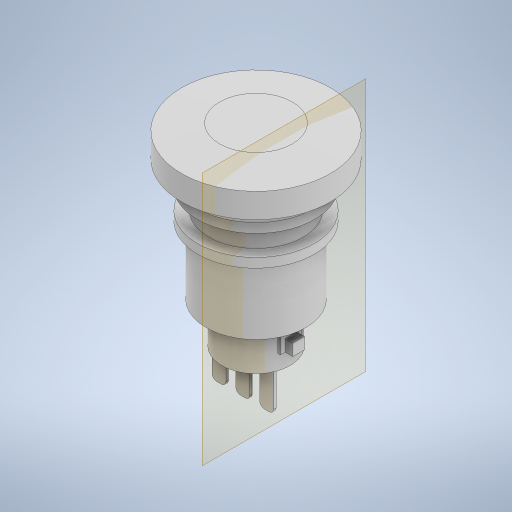
# Autodesk Inventor part: Co-1-01-eStopButton
Saved by Autodesk Inventor 2024 (Build 280153000, 153)
## iProperties
Created: 2023-02-23
Part Number: Co-1-01-eStopButton
Material: Generic
Document SubType Name: Modeling
Designer: t205b
Density: 1 g/cm^3
Appearance: Default
Author: t205b
Autodesk Inventor part; units mm, degrees
ref_plane "XZ Plane" through (0, 0, 0) normal (0, 1, 0) x (-1, 0, 0)
ref_plane "XY Plane" through (0, 0, 0) normal (0, 0, 1) x (1, 0, 0)
sketch "Sketch1" plane through (0, 0, 0) normal (0, 0, 1) x (1, 0, 0)
  line L0 (0, 20.0573) -> (0, -21.2213)
  line L1 (0, -21.2213) -> (-7.3, -21.2213)
  line L2 (-7.3, -21.2213) -> (-7.3, -12.5213)
  line L3 (-7.3, -12.5213) -> (-10.65, -12.5213)
  line L4 (-10.65, 1.9287) -> (-12.425, 1.9287)
  line L5 (-12.425, 1.9287) -> (-12.425, 3.9287)
  line L6 (-12.425, 3.9287) -> (-10.1, 3.9287)
  line L7 (-10.1, 3.9287) -> (-10.1, 8.4287)
  line L8 (-10.1, 8.4287) -> (-12.5, 8.4287)
  line L9 (-12.5, 8.4287) -> (-12.5, 10.4287)
  line L10 (-12.5, 10.4287) -> (-15.9, 13.3766)
  line L11 (-15.9, 13.3766) -> (-15.9, 18.6266)
  line L12 (0, 23.9493) -> (0, -31.6262)
  line L13 (-10.65, -12.5213) -> (-10.65, 1.9287)
  line L14 (-15.9, 18.6266) -> (-7.775, 20.0573)
  line L15 (-7.775, 20.0573) -> (0, 20.0573)
  point P0 (0, 0)
  point P1 (-10.1, 6.1787)
  point P2 (-10.65, -5.2963)
  dimension "d2" = 31.8
  dimension "d3" = 25
  dimension "d5" = 20.2
  dimension "d6" = 24.85
  dimension "d9" = 14.6
  dimension "d10" = 8.7
  dimension "d13" = 2
  dimension "d14" = 4.5
  dimension "d15" = 4.5
  dimension "d16" = 2
  dimension "d17" = 5.25
  dimension "d19" = 21.3
  dimension "d20" = 14.45
  dimension "d21" = 15.55
  dimension "d22" = 8.25
  constraints: 32 end point, 9 perpendicular, 3 point on line, 2 midpoint, 2 vertical, 1 parallel, 1 other
  measures "d2" diameter of L11 L12
  measures "d3" diameter of L9 L12
  measures "d5" diameter of L7 L12
  measures "d6" diameter of L5 L12
  measures "d9" diameter of L2 L12
  measures "d10" distance of L1.end L2.end
  measures "d13" distance of L4.end L5.end
  measures "d14" distance of L6.end L7.end
  measures "d15" distance of L9.end L10.end
  measures "d16" distance of L8.end L9.end
  measures "d17" distance of L10.end L11.end
  measures "d19" diameter of point (-10.65, -5.296) L12
  measures "d20" distance of L3.end L4.start
  measures "d21" diameter of L14.end L12
  measures "d22" distance of L11.end L14.end
revolve "Revolution1" add sketch "Sketch1" angle 360 about axis through (0, 23.9493, 0) along (0, -1, 0)
sketch "Sketch2" plane through (0, -21.2213, 0) normal (0, -1, 0) x (1, 0, 0)
  line L0 (6.6, 2.8) -> (3.6, 2.8)
  line L1 (3.6, 2.8) -> (3.6, 2.3)
  line L2 (3.6, 2.3) -> (6.6, 2.3)
  line L3 (6.6, 2.3) -> (6.6, 2.8)
  line L4 (1.5, 2.8) -> (-1.5, 2.8)
  line L5 (-1.5, 2.8) -> (-1.5, 2.3)
  line L6 (-1.5, 2.3) -> (1.5, 2.3)
  line L7 (1.5, 2.3) -> (1.5, 2.8)
  line L8 (-3.6, 2.8) -> (-6.6, 2.8)
  line L9 (-6.6, 2.8) -> (-6.6, 2.3)
  line L10 (-6.6, 2.3) -> (-3.6, 2.3)
  line L11 (-3.6, 2.3) -> (-3.6, 2.8)
  circle A0 centre (0, 0) radius 7.3 projected
  point P0 (0, 0)
  dimension "d23" = 0.5
  dimension "d24" = 3
  dimension "d25" = 2.1
  dimension "d26" = 2.1
  dimension "d29" = 14.6
  dimension "d31" = 2.8
  dimension "d32" = 1.5
  constraints: 24 end point, 6 parallel, 4 point on line, 3 horizontal, 3 perpendicular, 2 collinear
  measures "d23" distance of L0.end L1.end
  measures "d24" distance of L1.end L2.end
  measures "d25" distance between parallel lines of L1 L7
  measures "d26" distance between parallel lines of L5 L11
  measures "d29" diameter of A0
  measures "d31" distance from line of L4 A0.centre
  measures "d32" distance from line of point (0, 0) L7
extrude "Extrusion1" add sketch "Sketch2" along normal blind 8 contours L3 L2 L1 L0 | L7 L6 L5 L4 | L11 L10 L9 L8
fillet "Fillet1" radius 1 6 edges at (6.6, -29.2213, 2.55) (3.6, -29.2213, 2.55) (-6.6, -29.2213, 2.55) (-3.6, -29.2213, 2.55) (-1.5, -29.2213, 2.55) (1.5, -29.2213, 2.55)
ref_plane "Work Plane1" through (6, 0, 0) normal (1, 0, 0) x (0, 1, 0)
sketch "Sketch3" plane through (6, 0, 0) normal (1, 0, 0) x (0, 1, 0)
  line L0 (-12.5213, 7.3) -> (-12.5213, -7.3) projected
  line L1 (-12.5213, 2.25) -> (-18.0213, 2.25)
  line L2 (-18.0213, 2.25) -> (-18.0213, -2.25)
  line L3 (-18.0213, -2.25) -> (-12.5213, -2.25)
  line L4 (-12.5213, -2.25) -> (-12.5213, 2.25)
  line L5 (-39.077, 0) -> (29.913, 0) projected
  point P0 (0, 0)
  dimension "d37" = 4.5
  dimension "d38" = 5.5
  dimension "d39" = 2.25
  constraints: 8 end point, 2 parallel, 1 horizontal, 1 perpendicular, 1 point on line
  measures "d37" distance of L1.end L2.end
  measures "d38" distance of L2.end L3.end
  measures "d39" distance between parallel lines of L5 L3
extrude "Extrusion2" add sketch "Sketch3" along normal blind 1.5
sketch "Sketch4" plane through (7.5, 0, 0) normal (1, 0, 0) x (0, 0, -1)
  line L0 (-2.25, -18.0213) -> (2.25, -18.0213) projected
  line L1 (-1.25, -15.5213) -> (1.25, -15.5213)
  line L2 (1.25, -15.5213) -> (1.25, -18.0213)
  line L3 (1.25, -18.0213) -> (-1.25, -18.0213)
  line L4 (-1.25, -18.0213) -> (-1.25, -15.5213)
  line L5 (0, -39.077) -> (0, 29.913) projected
  point P0 (0, 0)
  dimension "d42" = 2.5
  dimension "d43" = 2.5
  dimension "d44" = 1.25
  constraints: 8 end point, 2 parallel, 1 horizontal, 1 perpendicular, 1 point on line
  measures "d42" distance of L1.end L2.end
  measures "d43" distance of L1.start L1.end
  measures "d44" distance between parallel lines of L5 L2
extrude "Extrusion3" add sketch "Sketch4" along normal blind 1.6
equation "\"d32\" = 0.5 * d24"
equation "\"d39\" = 0.5 * d37"
equation "\"d44\" = 0.5 * d43"
body "Solid1"
